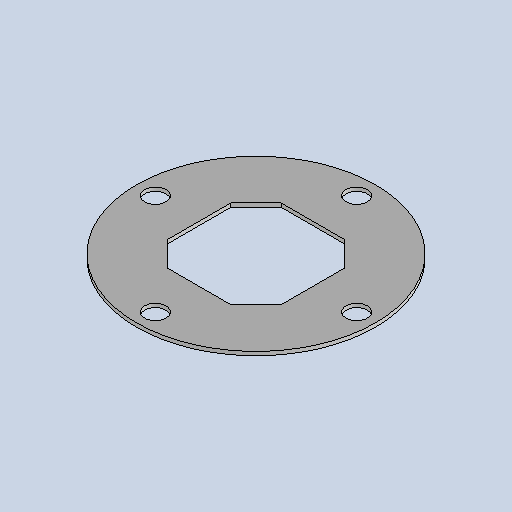
# Autodesk Inventor part: TZS 1651 FDS MAIN  FLANGE
Saved by Autodesk Inventor 2025.1 (Build 291241020, 241B)
## iProperties
Created: 2025-06-24
Part Number: TZS 1651 FDS MAIN  FLANGE
Material: Stainless Steel
Document SubType Name: Sheet Metal
Designer: admin
Mass: 483.479 g
Surface Area: 436.609 cm^2
Volume: 60.4349 cm^3
Density: 8 g/cm^3
Flat Pattern Width: 19 cm
Flat Pattern Length: 19 cm
Flat Pattern Area: 361 cm^2
Sheet Metal Rule: Default
Sheet Metal Width: 190.000 mm
Sheet Metal Length: 190.000 mm
Sheet Metal Area: 36100.000 mm^2
Appearance: Default
Author: user
Autodesk Inventor part; units mm, degrees
ref_plane "YZ Plane" through (0, 0, 0) normal (1, 0, 0) x (0, 1, 0)
ref_plane "XZ Plane" through (0, 0, 0) normal (0, 1, 0) x (-1, 0, 0)
ref_plane "XY Plane" through (0, 0, 0) normal (0, 0, 1) x (1, 0, 0)
sketch "Sketch1" plane through (0, 0, 0) normal (0, 0, 1) x (1, 0, 0)
  circle A0 centre (0, 0) radius 95
  line L0 (45, 45) -> (-45, 45)
  line L1 (-45, 45) -> (-45, -45)
  line L2 (-45, -45) -> (45, -45)
  line L3 (45, -45) -> (45, 45)
  line L4 (45, 45) -> (-45, -45) construction
  line L5 (-45, 45) -> (45, -45) construction
  dimension "d157" = 190
  dimension "d158" = 90
  dimension "d159" = 90
  measures "d157" diameter of A0
  measures "d158" distance of L2.end L1.end
  measures "d159" distance of L1.end L0.end
extrude "Plate5" add sketch "Sketch1" along normal blind 3
sketch "Sketch7" plane through (0, 0, 0) normal (0, 0, -1) x (-1, 0, 0)
  circle A0 centre (0, 80) radius 8.5
  point P0 (0, 0)
  dimension "d160" = 17
  dimension "d161" = 80
  constraints: 1 centre point, 1 vertical alignment
  measures "d160" diameter of A0
  measures "d161" distance of point (0, 0) A0.centre
extrude "Cut1" cut sketch "Sketch7" against normal blind 3
pattern_circular "Circular Pattern1" count 4 over 360 about axis through (0, 0, -10) along (0, 0, 1) of "Cut1"
chamfer "Corner Chamfer2" distance 20 angle 45 4 edges at (-45, -45, 1.5) (45, -45, 1.5) (-45, 45, 1.5) (45, 45, 1.5)
body "Solid3"
